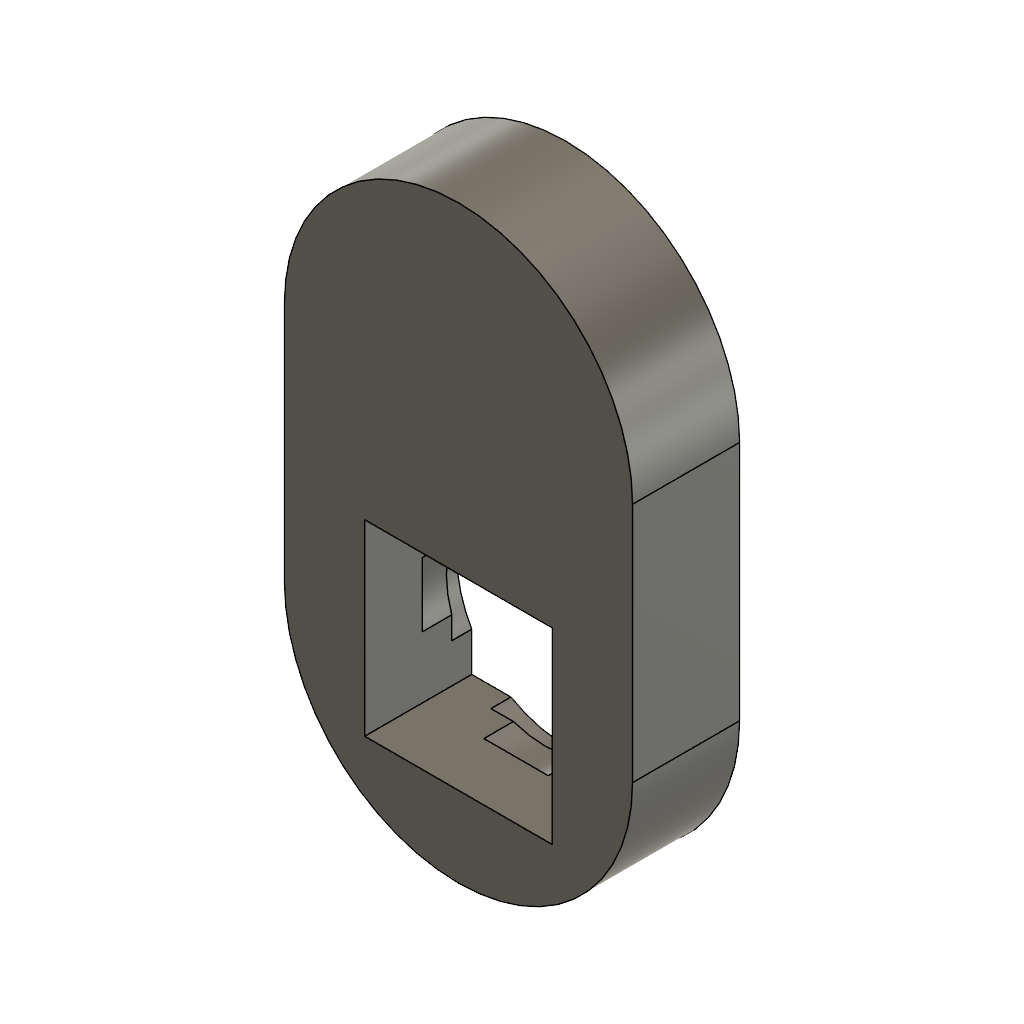
microscopio (Autodesk Fusion 360 design; units mm, degrees)
part number: 2026-09-25-17-02-42-894
Autodesk Fusion 360 part; units mm, degrees
note: some values were not read from the file. Set by a fixed rule: which sketch regions a step uses.
sketch "Boceto1" plane through (0, 0, 0) normal (0, 0, 1) x (1, 0, 0)
  circle A0 centre (0, 9) radius 13
  circle A1 centre (0, -9) radius 13
  line L0 (-13, -9) -> (-13, 9)
  line L1 (13, -9) -> (13, 9)
extrude "Extruir1" add sketch "Boceto1" along normal blind 8 makes body 1
sketch "Boceto2" plane through (0, 0, 0) normal (0, 0, 1) x (1, 0, 0)
  circle A0 centre (0, 9) radius 8.6
  circle A1 centre (0, -9) radius 8.6
  line L0 (-8.6, -9) -> (-8.6, 9)
  line L1 (8.6, -9) -> (8.6, 9)
extrude "Extruir2" cut sketch "Boceto2" along normal blind 1.5 bodies 1
sketch "Boceto3" plane through (0, 0, 0) normal (0, 0, 1) x (1, 0, 0)
  circle A0 centre (0, 9) radius 8.2
  circle A1 centre (0, -9) radius 8.2
extrude "Extruir3" cut sketch "Boceto3" along normal blind 3.7 bodies 1
sketch "Boceto4" plane through (0, 0, 0) normal (0, 0, 1) x (1, 0, 0)
  line L0 (-6.5, -15.5) -> (6.5, -15.5)
  line L1 (6.5, -15.5) -> (6.5, -2.5)
  line L2 (6.5, -2.5) -> (-6.5, -2.5)
  line L3 (-6.5, -2.5) -> (-6.5, -15.5)
extrude "Extruir4" cut sketch "Boceto4" along normal blind 8 bodies 1
sketch "Boceto5" plane through (0, 0, 0) normal (0, 0, 1) x (1, 0, 0)
  circle A0 centre (0, 9) radius 13
  circle A1 centre (0, -9) radius 13
  line L0 (-13, -9) -> (-13, 9)
  line L1 (13, -9) -> (13, 9)
extrude "Extruir5" add sketch "Boceto5" along normal blind 8 separate body makes body 2
sketch "Boceto6" plane through (0, 0, 0) normal (0, 0, 1) x (1, 0, 0)
  circle A0 centre (0, 9) radius 8.2
  circle A1 centre (0, -9) radius 8.2
  line L0 (-8.2, -9) -> (-8.2, 9)
  line L1 (8.2, -9) -> (8.2, 9)
extrude "Extruir6" cut sketch "Boceto6" along normal blind 1.5 bodies 2
sketch "Boceto7" plane through (0, 0, 0) normal (0, 0, 1) x (1, 0, 0)
  circle A0 centre (0, 9) radius 7.5
  circle A1 centre (0, -9) radius 7.5
extrude "Extruir7" cut sketch "Boceto7" along normal blind 3.7 bodies 2
sketch "Boceto8" plane through (0, 0, 0) normal (0, 0, 1) x (1, 0, 0)
  line L0 (-7, -16) -> (7, -16)
  line L1 (7, -16) -> (7, -2)
  line L2 (7, -2) -> (-7, -2)
  line L3 (-7, -2) -> (-7, -16)
extrude "Extruir8" cut sketch "Boceto8" along normal blind 8 bodies 2
sketch "Boceto9" plane through (0, 0, 0) normal (0, 0, 1) x (1, 0, 0)
  circle A0 centre (0, 9) radius 13
  circle A1 centre (0, -9) radius 13
  line L0 (-13, -9) -> (-13, 9)
  line L1 (13, -9) -> (13, 9)
extrude "Extruir9" add sketch "Boceto9" along normal blind 8 separate body makes body 3
sketch "Boceto10" plane through (0, 0, 0) normal (0, 0, 1) x (1, 0, 0)
  circle A0 centre (0, 9) radius 8.1
  circle A1 centre (0, -9) radius 8.1
  line L0 (-8.1, -9) -> (-8.1, 9)
  line L1 (8.1, -9) -> (8.1, 9)
extrude "Extruir10" cut sketch "Boceto10" along normal blind 1.5 bodies 3
sketch "Boceto11" plane through (0, 0, 0) normal (0, 0, 1) x (1, 0, 0)
  circle A0 centre (0, 9) radius 7.4
  circle A1 centre (0, -9) radius 7.4
extrude "Extruir11" cut sketch "Boceto11" along normal blind 3.7 bodies 3
sketch "Boceto12" plane through (0, 0, 0) normal (0, 0, 1) x (1, 0, 0)
  line L0 (-7, -16) -> (7, -16)
  line L1 (7, -16) -> (7, -2)
  line L2 (7, -2) -> (-7, -2)
  line L3 (-7, -2) -> (-7, -16)
extrude "Extruir12" cut sketch "Boceto12" along normal blind 8 bodies 3
hidden bodies 1 2
